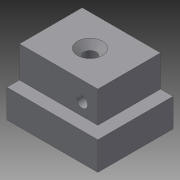
# Autodesk Inventor part: table_mount
Saved by Autodesk Inventor 2013 (Build 170138000, 138)
## iProperties
Created: 2014-02-26
Part Number: table_mount
Material: Ogólny
Document SubType Name: Modeling
Designer: Piotr
Density: 1 g/cm^3
Author: Piotr
Autodesk Inventor part; units mm, degrees
ref_plane "YZ Plane" through (0, 0, 0) normal (1, 0, 0) x (0, 1, 0)
ref_plane "XZ Plane" through (0, 0, 0) normal (0, 1, 0) x (-1, 0, 0)
ref_plane "XY Plane" through (0, 0, 0) normal (0, 0, 1) x (1, 0, 0)
sketch "Szkic1" plane through (0, 0, 0) normal (0, 0, 1) x (1, 0, 0)
  line L0 (-12.5, -10) -> (12.5, -10)
  line L1 (12.5, -10) -> (12.5, 10)
  line L2 (12.5, 10) -> (-12.5, 10)
  line L3 (-12.5, 10) -> (-12.5, -10)
  line L4 (-12.5, -10) -> (12.5, 10) construction
  line L5 (12.5, -10) -> (-12.5, 10) construction
  line L6 (-12.5, 10) -> (16.5, 10)
  line L7 (16.5, 10) -> (16.5, -14)
  line L8 (16.5, -14) -> (-12.5, -14)
  line L9 (-12.5, -14) -> (-12.5, 10)
  point P0 (0, 0)
  dimension "d0" = 25
  dimension "d1" = 20
  dimension "d2" = 4
  dimension "d3" = 4
  constraints: 20 end point, 4 parallel, 2 horizontal, 2 midpoint, 2 perpendicular
  measures "d0" distance of L2.end L1.end
  measures "d1" distance of L1.end L0.end
  measures "d2" distance between parallel lines of L0 L8
  measures "d3" distance between parallel lines of L7 L1
extrude "Wyciągnięcie proste1" add sketch "Szkic1" against normal blind 9
extrude "Wyciągnięcie proste2" add sketch "Szkic1" along normal blind 10 contours L3 L2 L1 L0
sketch "Szkic2" plane through (0, 0, 10) normal (0, 0, 1) x (1, 0, 0)
  point P0 (0, 0)
  point P1 (0, 0)
  constraints: 1 coincident
sketch "Szkic3" plane through (-12.5, -10, 0) normal (0, -1, 0) x (1, 0, 0)
  line L0 (25, 0) -> (0, 0) projected
  line L1 (25, 0) -> (25, 10) projected
  point P0 (12.5, 0)
  point P1 (20, 4)
  dimension "d8" = 5
  dimension "d9" = 4
  measures "d8" distance from line of L1 point (20, 4)
  measures "d9" distance from line of L0 point (20, 4)
hole "Otwór1" at (7.5, -10, 4) direction (0, 1, 0) diameter 3.5 end through all
hole "Otwór2" at (0, 0, 10) direction (0, 0, -1) diameter 4 end through all
chamfer "Faza1" distance 2 angle 45 1 edges at (0, 2, 10)
